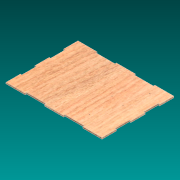
# Autodesk Inventor part: TAPA
Saved by Autodesk Inventor 2018 (Build 220112000, 112)
## iProperties
Created: 2019-12-06
Part Number: TAPA
Material: Generic
Document SubType Name: Modeling
Designer: Carlos Loaiza
Density: 1 g/cm^3
Appearance: Default
Author: Carlos Loaiza
Autodesk Inventor part; units mm, degrees
ref_plane "YZ Plane" through (0, 0, 0) normal (1, 0, 0) x (0, 1, 0)
ref_plane "XZ Plane" through (0, 0, 0) normal (0, 1, 0) x (-1, 0, 0)
ref_plane "XY Plane" through (0, 0, 0) normal (0, 0, 1) x (1, 0, 0)
sketch "Sketch1" plane through (0, 0, 0) normal (0, 0, 1) x (1, 0, 0)
  line L0 (0, 0) -> (200, 0)
  line L1 (200, 0) -> (200, 150)
  line L2 (200, 150) -> (0, 150)
  line L3 (0, 150) -> (0, 0)
  dimension "d0" = 200
  dimension "d1" = 150
  constraints: 8 end point, 2 perpendicular, 1 horizontal, 1 vertical
  measures "d0" distance of L0.start L0.end
  measures "d1" distance of L0.end L1.end
extrude "Extrusion1" add sketch "Sketch1" along normal blind 3
sketch "Sketch2" plane through (0, 0, 3) normal (0, 0, 1) x (1, 0, 0)
  line L0 (0, 0) -> (40, 0)
  line L1 (0, 0) -> (200, 0) projected
  line L2 (40, 0) -> (40, 3)
  line L3 (40, 3) -> (80, 3)
  line L4 (80, 3) -> (80, 0)
  line L5 (80, 0) -> (120, 0)
  line L6 (0, 150) -> (0, 0) projected
  line L7 (0, 75) -> (200, 75)
  line L8 (200, 0) -> (200, 150) projected
  line L9 (120, 0) -> (120, 3)
  line L10 (120, 3) -> (160, 3)
  line L11 (160, 3) -> (160, 0)
  line L12 (40, 0) -> (80, 0)
  line L13 (120, 0) -> (160, 0)
  line L14 (200, 150) -> (0, 150) projected
  line L15 (0, 150) -> (0, 120)
  line L16 (0, 120) -> (3, 120)
  line L17 (3, 120) -> (3, 90)
  line L18 (3, 90) -> (0, 90)
  line L19 (0, 90) -> (0, 60)
  line L20 (0, 60) -> (3, 60)
  line L21 (3, 60) -> (3, 30)
  line L22 (3, 30) -> (0, 30)
  line L23 (0, 30) -> (0, 0)
  line L24 (100, 150) -> (100, 0)
  line L25 (0, 60) -> (0, 30)
  line L26 (0, 120) -> (0, 90)
  line L27 (200, 120) -> (197, 120)
  line L28 (197, 120) -> (197, 90)
  line L29 (197, 90) -> (200, 90)
  line L30 (200, 90) -> (200, 60)
  line L31 (200, 60) -> (197, 60)
  line L32 (197, 60) -> (197, 30)
  line L33 (197, 30) -> (200, 30)
  line L34 (200, 60) -> (200, 30)
  line L35 (200, 120) -> (200, 90)
  line L36 (40, 150) -> (40, 147)
  line L37 (40, 147) -> (80, 147)
  line L38 (80, 147) -> (80, 150)
  line L39 (80, 150) -> (120, 150)
  line L40 (120, 150) -> (120, 147)
  line L41 (120, 147) -> (160, 147)
  line L42 (160, 147) -> (160, 150)
  line L43 (40, 150) -> (80, 150)
  line L44 (120, 150) -> (160, 150)
  dimension "d4" = 40
  dimension "d6" = 3
  dimension "d7" = 40
  dimension "d8" = 40
  dimension "d19" = 40
  dimension "d20" = 30
  dimension "d21" = 3
  dimension "d22" = 30
  dimension "d23" = 30
  dimension "d24" = 30
  constraints: 82 end point, 16 symmetric about line, 12 point on line, 9 perpendicular, 4 collinear, 4 midpoint, 2 vertical, 1 horizontal
  measures "d4" distance of L0.start L0.end
  measures "d6" distance of L0.end L2.end
  measures "d7" distance of L2.end L3.end
  measures "d8" distance of L4.end L5.end
  measures "d19" distance of L9.end L10.end
  measures "d20" distance of L6.start L15.end
  measures "d21" distance of L15.end L16.end
  measures "d22" distance of L16.end L17.end
  measures "d23" distance of L18.end L19.end
  measures "d24" distance of L20.end L21.end
extrude "Extrusion2" cut sketch "Sketch2" against normal blind 3 contours L2 L3 L4 L1 | L6 L20 L21 L22 | L9 L10 L11 L1 | L6 L16 L17 L18 | L8 L33 L32 L31 | L29 L28 L27 L8 | L14 L42 L41 L40 | L38 L37 L36 L14
body "Solid1"
